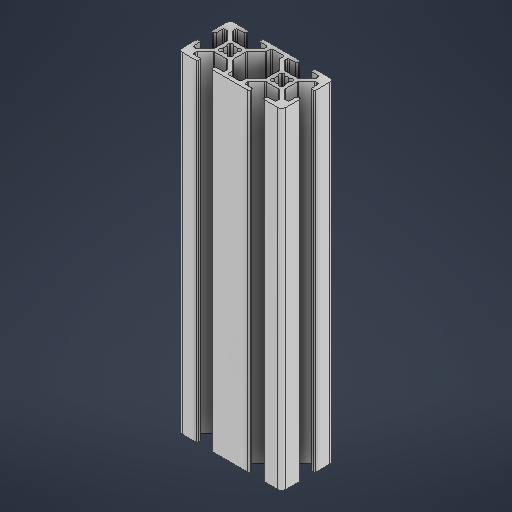
# Autodesk Inventor part: 20x40x128mm-Extrusion
Saved by Autodesk Inventor 2026.2 (Build 302298000, 298)
## iProperties
Created: 2026-06-17
Part Number: 20x40x128mm-Extrusion
Material: Aluminum 6061
Document SubType Name: Modeling
Designer: Kenji
Density: 2.7 g/cm^3
Appearance: Aluminum - Dark
Author: Kenji
Autodesk Inventor part; units mm, degrees
ref_plane "YZ Plane" through (0, 0, 0) normal (1, 0, 0) x (0, 1, 0)
ref_plane "XZ Plane" through (0, 0, 0) normal (0, 1, 0) x (-1, 0, 0)
ref_plane "XY Plane" through (0, 0, 0) normal (0, 0, 1) x (1, 0, 0)
sketch "Sketch1" plane through (0, 0, 0) normal (0, 1, 0) x (-1, 0, 0)
  arc A0 (12.7041, -3.8233) -> (12.3449, -3.6745) centre (12.3449, -4.1825) ccw
  line L0 (15.8072, -6.9264) -> (12.7041, -3.8233)
  arc A1 (15.956, -7.2856) -> (15.8072, -6.9264) centre (15.448, -7.2856) ccw
  line L1 (15.956, -8.0115) -> (15.956, -7.2856)
  arc A2 (15.448, -8.5195) -> (15.956, -8.0115) centre (15.448, -8.0115) ccw
  line L2 (13.099, -8.5195) -> (15.448, -8.5195)
  arc A3 (13.099, -8.5195) -> (12.591, -9.0275) centre (13.099, -9.0275) ccw
  line L3 (12.591, -9.5115) -> (12.591, -9.0275)
  arc A4 (12.591, -9.5115) -> (13.099, -10.0195) centre (13.099, -9.5115) ccw
  line L4 (18.461, -10.0195) -> (13.099, -10.0195)
  arc A5 (18.461, -10.0195) -> (19.961, -8.5195) centre (18.461, -8.5195) ccw
  line L5 (19.961, -3.1575) -> (19.961, -8.5195)
  arc A6 (19.961, -3.1575) -> (19.453, -2.6495) centre (19.453, -3.1575) ccw
  line L6 (18.969, -2.6495) -> (19.453, -2.6495)
  arc A7 (18.969, -2.6495) -> (18.461, -3.1575) centre (18.969, -3.1575) ccw
  line L7 (18.461, -5.5065) -> (18.461, -3.1575)
  arc A8 (17.953, -6.0145) -> (18.461, -5.5065) centre (17.953, -5.5065) ccw
  line L8 (17.2271, -6.0145) -> (17.953, -6.0145)
  arc A9 (16.8679, -5.8657) -> (17.2271, -6.0145) centre (17.2271, -5.5065) ccw
  line L9 (13.7648, -2.7626) -> (16.8679, -5.8657)
  arc A10 (13.616, -2.4034) -> (13.7648, -2.7626) centre (14.124, -2.4034) ccw
  line L10 (13.616, 2.3644) -> (13.616, -2.4034)
  arc A11 (13.7648, 2.7236) -> (13.616, 2.3644) centre (14.124, 2.3644) ccw
  line L11 (16.8679, 5.8267) -> (13.7648, 2.7236)
  arc A12 (17.2271, 5.9755) -> (16.8679, 5.8267) centre (17.2271, 5.4675) ccw
  line L12 (17.953, 5.9755) -> (17.2271, 5.9755)
  arc A13 (18.461, 5.4675) -> (17.953, 5.9755) centre (17.953, 5.4675) ccw
  line L13 (18.461, 3.1185) -> (18.461, 5.4675)
  arc A14 (18.461, 3.1185) -> (18.969, 2.6105) centre (18.969, 3.1185) ccw
  line L14 (19.453, 2.6105) -> (18.969, 2.6105)
  arc A15 (19.453, 2.6105) -> (19.961, 3.1185) centre (19.453, 3.1185) ccw
  line L15 (19.961, 8.4805) -> (19.961, 3.1185)
  arc A16 (19.961, 8.4805) -> (18.461, 9.9805) centre (18.461, 8.4805) ccw
  line L16 (13.099, 9.9805) -> (18.461, 9.9805)
  arc A17 (13.099, 9.9805) -> (12.591, 9.4725) centre (13.099, 9.4725) ccw
  line L17 (12.591, 8.9885) -> (12.591, 9.4725)
  arc A18 (12.591, 8.9885) -> (13.099, 8.4805) centre (13.099, 8.9885) ccw
  line L18 (15.448, 8.4805) -> (13.099, 8.4805)
  arc A19 (15.956, 7.9725) -> (15.448, 8.4805) centre (15.448, 7.9725) ccw
  line L19 (15.956, 7.2466) -> (15.956, 7.9725)
  arc A20 (15.8072, 6.8874) -> (15.956, 7.2466) centre (15.448, 7.2466) ccw
  line L20 (12.7041, 3.7843) -> (15.8072, 6.8874)
  arc A21 (12.3449, 3.6355) -> (12.7041, 3.7843) centre (12.3449, 4.1435) ccw
  line L21 (7.5771, 3.6355) -> (12.3449, 3.6355)
  arc A22 (7.2179, 3.7843) -> (7.5771, 3.6355) centre (7.5771, 4.1435) ccw
  line L22 (4.1148, 6.8874) -> (7.2179, 3.7843)
  arc A23 (3.966, 7.2466) -> (4.1148, 6.8874) centre (4.474, 7.2466) ccw
  line L23 (3.966, 7.9725) -> (3.966, 7.2466)
  arc A24 (4.474, 8.4805) -> (3.966, 7.9725) centre (4.474, 7.9725) ccw
  line L24 (6.823, 8.4805) -> (4.474, 8.4805)
  arc A25 (6.823, 8.4805) -> (7.331, 8.9885) centre (6.823, 8.9885) ccw
  line L25 (7.331, 9.4725) -> (7.331, 8.9885)
  arc A26 (7.331, 9.4725) -> (6.823, 9.9805) centre (6.823, 9.4725) ccw
  line L26 (-6.901, 9.9805) -> (6.823, 9.9805)
  arc A27 (-6.901, 9.9805) -> (-7.409, 9.4725) centre (-6.901, 9.4725) ccw
  line L27 (-7.409, 8.9885) -> (-7.409, 9.4725)
  arc A28 (-7.409, 8.9885) -> (-6.901, 8.4805) centre (-6.901, 8.9885) ccw
  line L28 (-4.552, 8.4805) -> (-6.901, 8.4805)
  arc A29 (-4.044, 7.9725) -> (-4.552, 8.4805) centre (-4.552, 7.9725) ccw
  line L29 (-4.044, 7.2466) -> (-4.044, 7.9725)
  arc A30 (-4.1928, 6.8874) -> (-4.044, 7.2466) centre (-4.552, 7.2466) ccw
  line L30 (-7.2959, 3.7843) -> (-4.1928, 6.8874)
  arc A31 (-7.6551, 3.6355) -> (-7.2959, 3.7843) centre (-7.6551, 4.1435) ccw
  line L31 (-12.4229, 3.6355) -> (-7.6551, 3.6355)
  arc A32 (-12.7821, 3.7843) -> (-12.4229, 3.6355) centre (-12.4229, 4.1435) ccw
  line L32 (-15.8852, 6.8874) -> (-12.7821, 3.7843)
  arc A33 (-16.034, 7.2466) -> (-15.8852, 6.8874) centre (-15.526, 7.2466) ccw
  line L33 (-16.034, 7.9725) -> (-16.034, 7.2466)
  arc A34 (-15.526, 8.4805) -> (-16.034, 7.9725) centre (-15.526, 7.9725) ccw
  line L34 (-13.177, 8.4805) -> (-15.526, 8.4805)
  arc A35 (-13.177, 8.4805) -> (-12.669, 8.9885) centre (-13.177, 8.9885) ccw
  line L35 (-12.669, 9.4725) -> (-12.669, 8.9885)
  arc A36 (-12.669, 9.4725) -> (-13.177, 9.9805) centre (-13.177, 9.4725) ccw
  line L36 (-18.539, 9.9805) -> (-13.177, 9.9805)
  arc A37 (-18.539, 9.9805) -> (-20.039, 8.4805) centre (-18.539, 8.4805) ccw
  line L37 (-20.039, 3.1185) -> (-20.039, 8.4805)
  arc A38 (-20.039, 3.1185) -> (-19.531, 2.6105) centre (-19.531, 3.1185) ccw
  line L38 (-19.047, 2.6105) -> (-19.531, 2.6105)
  arc A39 (-19.047, 2.6105) -> (-18.539, 3.1185) centre (-19.047, 3.1185) ccw
  line L39 (-18.539, 5.4675) -> (-18.539, 3.1185)
  arc A40 (-18.031, 5.9755) -> (-18.539, 5.4675) centre (-18.031, 5.4675) ccw
  line L40 (-17.3051, 5.9755) -> (-18.031, 5.9755)
  arc A41 (-16.9459, 5.8267) -> (-17.3051, 5.9755) centre (-17.3051, 5.4675) ccw
  line L41 (-13.8428, 2.7236) -> (-16.9459, 5.8267)
  arc A42 (-13.694, 2.3644) -> (-13.8428, 2.7236) centre (-14.202, 2.3644) ccw
  line L42 (-13.694, -2.4034) -> (-13.694, 2.3644)
  arc A43 (-13.8428, -2.7626) -> (-13.694, -2.4034) centre (-14.202, -2.4034) ccw
  line L43 (-16.9459, -5.8657) -> (-13.8428, -2.7626)
  arc A44 (-17.3051, -6.0145) -> (-16.9459, -5.8657) centre (-17.3051, -5.5065) ccw
  line L44 (-18.031, -6.0145) -> (-17.3051, -6.0145)
  arc A45 (-18.539, -5.5065) -> (-18.031, -6.0145) centre (-18.031, -5.5065) ccw
  line L45 (-18.539, -3.1575) -> (-18.539, -5.5065)
  arc A46 (-18.539, -3.1575) -> (-19.047, -2.6495) centre (-19.047, -3.1575) ccw
  line L46 (-19.531, -2.6495) -> (-19.047, -2.6495)
  arc A47 (-19.531, -2.6495) -> (-20.039, -3.1575) centre (-19.531, -3.1575) ccw
  line L47 (-20.039, -8.5195) -> (-20.039, -3.1575)
  arc A48 (-20.039, -8.5195) -> (-18.539, -10.0195) centre (-18.539, -8.5195) ccw
  line L48 (-13.177, -10.0195) -> (-18.539, -10.0195)
  arc A49 (-13.177, -10.0195) -> (-12.669, -9.5115) centre (-13.177, -9.5115) ccw
  line L49 (-12.669, -9.0275) -> (-12.669, -9.5115)
  arc A50 (-12.669, -9.0275) -> (-13.177, -8.5195) centre (-13.177, -9.0275) ccw
  line L50 (-15.526, -8.5195) -> (-13.177, -8.5195)
  arc A51 (-16.034, -8.0115) -> (-15.526, -8.5195) centre (-15.526, -8.0115) ccw
  line L51 (-16.034, -7.2856) -> (-16.034, -8.0115)
  arc A52 (-15.8852, -6.9264) -> (-16.034, -7.2856) centre (-15.526, -7.2856) ccw
  line L52 (-12.7821, -3.8233) -> (-15.8852, -6.9264)
  arc A53 (-12.4229, -3.6745) -> (-12.7821, -3.8233) centre (-12.4229, -4.1825) ccw
  line L53 (-7.6551, -3.6745) -> (-12.4229, -3.6745)
  arc A54 (-7.2959, -3.8233) -> (-7.6551, -3.6745) centre (-7.6551, -4.1825) ccw
  line L54 (-4.1928, -6.9264) -> (-7.2959, -3.8233)
  arc A55 (-4.044, -7.2856) -> (-4.1928, -6.9264) centre (-4.552, -7.2856) ccw
  line L55 (-4.044, -8.0115) -> (-4.044, -7.2856)
  arc A56 (-4.552, -8.5195) -> (-4.044, -8.0115) centre (-4.552, -8.0115) ccw
  line L56 (-6.901, -8.5195) -> (-4.552, -8.5195)
  arc A57 (-6.901, -8.5195) -> (-7.409, -9.0275) centre (-6.901, -9.0275) ccw
  line L57 (-7.409, -9.5115) -> (-7.409, -9.0275)
  arc A58 (-7.409, -9.5115) -> (-6.901, -10.0195) centre (-6.901, -9.5115) ccw
  line L58 (6.823, -10.0195) -> (-6.901, -10.0195)
  arc A59 (6.823, -10.0195) -> (7.331, -9.5115) centre (6.823, -9.5115) ccw
  line L59 (7.331, -9.0275) -> (7.331, -9.5115)
  arc A60 (7.331, -9.0275) -> (6.823, -8.5195) centre (6.823, -9.0275) ccw
  line L60 (4.474, -8.5195) -> (6.823, -8.5195)
  arc A61 (3.966, -8.0115) -> (4.474, -8.5195) centre (4.474, -8.0115) ccw
  line L61 (3.966, -7.2856) -> (3.966, -8.0115)
  arc A62 (4.1148, -6.9264) -> (3.966, -7.2856) centre (4.474, -7.2856) ccw
  line L62 (7.2179, -3.8233) -> (4.1148, -6.9264)
  arc A63 (7.5771, -3.6745) -> (7.2179, -3.8233) centre (7.5771, -4.1825) ccw
  line L63 (12.3449, -3.6745) -> (7.5771, -3.6745)
  arc A64 (-9.235, -1.9546) -> (-7.9141, -2.324) centre (-8.4706, -1.7675) ccw
  arc A65 (-10.843, -1.9546) -> (-9.235, -1.9546) centre (-10.039, -0.0195) ccw
  arc A66 (-12.1639, -2.324) -> (-10.843, -1.9546) centre (-11.6074, -1.7675) ccw
  line L64 (-12.1639, -2.324) -> (-12.3435, -2.1444)
  arc A67 (-11.9741, -0.8235) -> (-12.3435, -2.1444) centre (-11.787, -1.5879) ccw
  arc A68 (-11.9741, 0.7845) -> (-11.9741, -0.8235) centre (-10.039, -0.0195) ccw
  arc A69 (-12.3435, 2.1054) -> (-11.9741, 0.7845) centre (-11.787, 1.5489) ccw
  line L65 (-12.3435, 2.1054) -> (-12.1639, 2.285)
  arc A70 (-10.843, 1.9156) -> (-12.1639, 2.285) centre (-11.6074, 1.7285) ccw
  arc A71 (-9.235, 1.9156) -> (-10.843, 1.9156) centre (-10.039, -0.0195) ccw
  arc A72 (-7.9141, 2.285) -> (-9.235, 1.9156) centre (-8.4706, 1.7285) ccw
  line L66 (-7.9141, 2.285) -> (-7.7345, 2.1054)
  arc A73 (-8.1039, 0.7845) -> (-7.7345, 2.1054) centre (-8.291, 1.5489) ccw
  arc A74 (-8.1039, -0.8235) -> (-8.1039, 0.7845) centre (-10.039, -0.0195) ccw
  arc A75 (-7.7345, -2.1444) -> (-8.1039, -0.8235) centre (-8.291, -1.5879) ccw
  line L67 (-7.7345, -2.1444) -> (-7.9141, -2.324)
  arc A76 (10.765, -1.9546) -> (12.0859, -2.324) centre (11.5294, -1.7675) ccw
  arc A77 (9.157, -1.9546) -> (10.765, -1.9546) centre (9.961, -0.0195) ccw
  arc A78 (7.8361, -2.324) -> (9.157, -1.9546) centre (8.3926, -1.7675) ccw
  line L68 (7.8361, -2.324) -> (7.6565, -2.1444)
  arc A79 (8.0259, -0.8235) -> (7.6565, -2.1444) centre (8.213, -1.5879) ccw
  arc A80 (8.0259, 0.7845) -> (8.0259, -0.8235) centre (9.961, -0.0195) ccw
  arc A81 (7.6565, 2.1054) -> (8.0259, 0.7845) centre (8.213, 1.5489) ccw
  line L69 (7.6565, 2.1054) -> (7.8361, 2.285)
  arc A82 (9.157, 1.9156) -> (7.8361, 2.285) centre (8.3926, 1.7285) ccw
  arc A83 (10.765, 1.9156) -> (9.157, 1.9156) centre (9.961, -0.0195) ccw
  arc A84 (12.0859, 2.285) -> (10.765, 1.9156) centre (11.5294, 1.7285) ccw
  line L70 (12.0859, 2.285) -> (12.2655, 2.1054)
  arc A85 (11.8961, 0.7845) -> (12.2655, 2.1054) centre (11.709, 1.5489) ccw
  arc A86 (11.8961, -0.8235) -> (11.8961, 0.7845) centre (9.961, -0.0195) ccw
  arc A87 (12.2655, -2.1444) -> (11.8961, -0.8235) centre (11.709, -1.5879) ccw
  line L71 (12.2655, -2.1444) -> (12.0859, -2.324)
  arc A88 (1.958, -8.5195) -> (2.466, -8.0115) centre (1.958, -8.0115) ccw
  line L72 (1.958, -8.5195) -> (-2.036, -8.5195)
  arc A89 (-2.544, -8.0115) -> (-2.036, -8.5195) centre (-2.036, -8.0115) ccw
  line L73 (-2.544, -8.0115) -> (-2.544, -6.6643)
  arc A90 (-2.544, -6.6643) -> (-2.6928, -6.305) centre (-3.052, -6.6643) ccw
  line L74 (-2.6928, -6.305) -> (-6.2352, -2.7626)
  arc A91 (-6.384, -2.4034) -> (-6.2352, -2.7626) centre (-5.876, -2.4034) ccw
  line L75 (-6.384, -2.4034) -> (-6.384, 2.3644)
  arc A92 (-6.2352, 2.7236) -> (-6.384, 2.3644) centre (-5.876, 2.3644) ccw
  line L76 (-6.2352, 2.7236) -> (-2.6928, 6.2661)
  arc A93 (-2.6928, 6.2661) -> (-2.544, 6.6253) centre (-3.052, 6.6253) ccw
  line L77 (-2.544, 6.6253) -> (-2.544, 7.9725)
  arc A94 (-2.036, 8.4805) -> (-2.544, 7.9725) centre (-2.036, 7.9725) ccw
  line L78 (-2.036, 8.4805) -> (1.958, 8.4805)
  arc A95 (2.466, 7.9725) -> (1.958, 8.4805) centre (1.958, 7.9725) ccw
  line L79 (2.466, 7.9725) -> (2.466, 6.6253)
  arc A96 (2.466, 6.6253) -> (2.6148, 6.2661) centre (2.974, 6.6253) ccw
  line L80 (2.6148, 6.2661) -> (6.1572, 2.7236)
  arc A97 (6.306, 2.3644) -> (6.1572, 2.7236) centre (5.798, 2.3644) ccw
  line L81 (6.306, 2.3644) -> (6.306, -2.4034)
  arc A98 (6.1572, -2.7626) -> (6.306, -2.4034) centre (5.798, -2.4034) ccw
  line L82 (6.1572, -2.7626) -> (2.6148, -6.305)
  arc A99 (2.6148, -6.305) -> (2.466, -6.6643) centre (2.974, -6.6643) ccw
  line L83 (2.466, -6.6643) -> (2.466, -8.0115)
  point P0 (0, 0)
  constraints: 200 point on circle, 168 end point, 100 centre point, 32 vertical, 28 horizontal, 409 other
extrude "Extrusion1" add sketch "Sketch1" along normal blind 128
body "Solid1"
